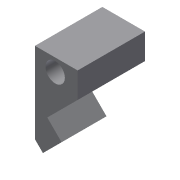
# Autodesk Inventor part: TensionMountV2
Saved by Autodesk Inventor 2013 (Build 170138000, 138)
## iProperties
Created: 2014-12-18
Part Number: TensionMountV2
Material: Generic
Document SubType Name: Modeling
Designer: 120pa
Density: 1 g/cm^3
Author: 120pa
Autodesk Inventor part; units mm, degrees
ref_plane "YZ Plane" through (0, 0, 0) normal (1, 0, 0) x (0, 1, 0)
ref_plane "XZ Plane" through (0, 0, 0) normal (0, 1, 0) x (-1, 0, 0)
ref_plane "XY Plane" through (0, 0, 0) normal (0, 0, 1) x (1, 0, 0)
sketch "Sketch1" plane through (0, 0, 0) normal (0, 1, 0) x (-1, 0, 0)
  line L0 (0, -5.6886) -> (6.7556, -12.4442)
  line L1 (6.7556, -12.4442) -> (5.3414, -13.8584)
  line L2 (9.5, -18.017) -> (5.3414, -13.8584)
  line L3 (10, -18.017) -> (9.5, -18.017)
  line L4 (10, -18.017) -> (10, 0)
  line L5 (0, 0) -> (10, 0)
  line L6 (0, 0) -> (0, -5.6886)
  circle A0 centre (5, -2.8443) radius 1.339
  constraints: 14 end point, 1 centre point
extrude "Extrusion1" add sketch "Sketch1" along normal blind 10
sketch "Sketch2" plane through (0, 10, 0) normal (0, 1, 0) x (1, 0, 0)
  line L0 (0, 5.6886) -> (-10, 5.6886)
  line L1 (-10, 5.6886) -> (-10, 0)
  line L2 (-10, 0) -> (0, 0)
  line L3 (0, 0) -> (0, 5.6886)
  constraints: 8 end point
extrude "Extrusion2" add sketch "Sketch2" along normal blind 20
sketch "Sketch3" plane through (0, 0, 0) normal (0, -1, 0) x (1, 0, 0)
  circle A0 centre (-5, -2.8443) radius 1.339 projected
hole "Hole1" at (-5, 0, -2.8443) direction (0, 1, 0) diameter 4.318 end through all
sketch "Sketch8" plane through (-9.5, 0, -18.017) normal (0.7071068, 0, -0.7071068) x (-0.7071068, 0, -0.7071068)
  line L0 (-5.8811, 0) -> (0, 0) projected
  line L1 (0, 0) -> (0, 10) projected
  line L2 (-5.8811, 10) -> (0, 10) projected
  line L3 (-5.8811, 0) -> (-5.8811, 10) projected
  line L4 (-1.0406, 1) -> (-4.8406, 1)
  line L5 (-4.8406, 1) -> (-4.8406, 9)
  line L6 (-4.8406, 9) -> (-1.0406, 9)
  line L7 (-1.0406, 9) -> (-1.0406, 1)
  line L8 (-1.0406, 1) -> (-4.8406, 9) construction
  line L9 (-4.8406, 1) -> (-1.0406, 9) construction
  point P0 (-19.4575, 0)
  point P1 (-2.9406, 5)
  dimension "d41" = 3.8
  dimension "d42" = 8
  constraints: 12 end point, 2 midpoint
  measures "d41" distance of L5.end L6.end
  measures "d42" distance of L4.end L5.end
extrude "Extrusion6" add sketch "Sketch8" along normal blind 2.5
sketch "Sketch9" plane through (-6.0772, 1, -14.5942) normal (-0.7071068, 0, -0.7071068) x (-0.7071068, 0, 0.7071068)
  line L0 (-2.25, 7) -> (-1.75, 7)
  line L1 (-1.75, 7) -> (-1.75, 6.5)
  line L2 (-1.75, 6.5) -> (-2.25, 6.5)
  line L3 (-2.25, 6.5) -> (-2.25, 7)
  line L4 (-1.75, 1) -> (-2.25, 1)
  line L5 (-2.25, 1) -> (-2.25, 1.5)
  line L6 (-2.25, 1.5) -> (-1.75, 1.5)
  line L7 (-1.75, 1.5) -> (-1.75, 1)
  point P0 (6.0224, -1)
  dimension "d45" = 0.5
  dimension "d46" = 0.5
  dimension "d47" = 0.5
  dimension "d48" = 0.5
  constraints: 16 end point
  measures "d45" distance of L1.end L2.end
  measures "d46" distance of L0.end L1.end
  measures "d47" distance of L5.end L6.end
  measures "d48" distance of L4.end L5.end
extrude "Extrusion7" add sketch "Sketch9" along normal blind 4
sketch "Sketch10" plane through (0, 30, 0) normal (0, 1, 0) x (1, 0, 0)
  circle A0 centre (-5, 2.8443) radius 2.159 projected
  line L0 (0, 5.6886) -> (-10, 5.6886) projected
  line L1 (-10, 5.6886) -> (-10, 0) projected
  line L2 (-10, 0) -> (0, 0) projected
  line L3 (0, 0) -> (0, 5.6886) projected
extrude "Extrusion8" cut sketch "Sketch10" against normal blind 15
sketch "Sketch11" plane through (-10, 0, -18.017) normal (-1, 0, 0) x (0, 0, 1)
  line L0 (18.017, 15) -> (12.3284, 15) projected
  line L1 (12.3284, 10) -> (12.3284, 15) projected
  line L2 (0, 10) -> (12.3284, 10) projected
  line L3 (0, 0) -> (0, 10) projected
  line L4 (0, 0) -> (18.017, 0) projected
  line L5 (18.017, 0) -> (18.017, 15) projected
extrude "Extrusion9" cut sketch "Sketch11" against normal blind 0.5
body "Solid1"
